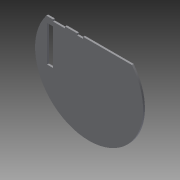
# Autodesk Inventor part: Base Plate
Saved by Autodesk Inventor 2015 (Build 190159000, 159)
## iProperties
Created: 2014-11-10
Part Number: Base Plate
Material: Generic
Document SubType Name: Modeling
Designer: karl
Density: 1 g/cm^3
Appearance: Default
Author: karl
Autodesk Inventor part; units mm, degrees
ref_plane "YZ Plane" through (0, 0, 0) normal (1, 0, 0) x (0, 1, 0)
ref_plane "XZ Plane" through (0, 0, 0) normal (0, 1, 0) x (-1, 0, 0)
ref_plane "XY Plane" through (0, 0, 0) normal (0, 0, 1) x (1, 0, 0)
sketch "Sketch1" plane through (0, 0, 0) normal (0, 1, 0) x (-1, 0, 0)
  circle A0 centre (0, 0) radius 90
  line L0 (-71.239, 55) -> (71.239, 55)
  dimension "d0" = 180
  dimension "d1" = 55
  constraints: 2 end point, 2 point on circle, 1 centre point, 1 coincident, 1 horizontal
  measures "d0" diameter of A0
  measures "d1" distance from line of point (0, 0) L0
extrude "Extrusion1" add sketch "Sketch1" along normal blind 3 contours A0 L0 picked at (-1.0947, 6.6866)
sketch "Sketch2" plane through (0, 3, 0) normal (0, 1, 0) x (1, 0, 0)
  line L0 (-70, -45) -> (-60, -45)
  line L1 (-60, -45) -> (-60, 15)
  line L2 (-60, 15) -> (-70, 15)
  line L3 (-70, 15) -> (-70, -45)
  line L4 (-70, -45) -> (-60, 15) construction
  line L5 (-60, -45) -> (-70, 15) construction
  point P0 (0, 0)
  point P1 (-65, -15)
  dimension "d4" = 10
  dimension "d5" = 60
  dimension "d6" = 15
  dimension "d7" = 65
  constraints: 12 end point, 2 midpoint, 2 parallel, 1 horizontal, 1 perpendicular
  measures "d4" distance of L2.end L1.end
  measures "d5" distance of L1.end L0.end
  measures "d6" vertical distance of point (0, 0) point (-65, -15)
  measures "d7" horizontal distance of point (0, 0) point (-65, -15)
extrude "Extrusion2" cut sketch "Sketch2" against normal blind 3
sketch "Sketch3" plane through (0, 3, 0) normal (0, 1, 0) x (1, 0, 0)
  line L0 (-71.239, -55) -> (71.239, -55) projected
  line L1 (-60, -55) -> (-40, -55)
  line L2 (-40, -55) -> (-40, -52)
  line L3 (-40, -52) -> (-60, -52)
  line L4 (-60, -52) -> (-60, -55)
  line L5 (-20, -55) -> (-10, -55)
  line L6 (-10, -55) -> (-10, -52)
  line L7 (-10, -52) -> (-20, -52)
  line L8 (-20, -52) -> (-20, -55)
  point P0 (0, 0)
  dimension "d10" = 20
  dimension "d11" = 3
  dimension "d12" = 10
  dimension "d13" = 3
  dimension "d14" = 10
  dimension "d15" = 20
  constraints: 16 end point, 4 parallel, 2 horizontal, 2 perpendicular, 2 point on line
  measures "d10" distance of L3.end L2.end
  measures "d11" distance of L2.end L1.end
  measures "d12" distance of L7.end L6.end
  measures "d13" distance of L6.end L5.end
  measures "d14" distance from line of point (0, 0) L6
  measures "d15" distance between parallel lines of L8 L2
extrude "Extrusion3" cut sketch "Sketch3" against normal blind 3
body "Solid1"
